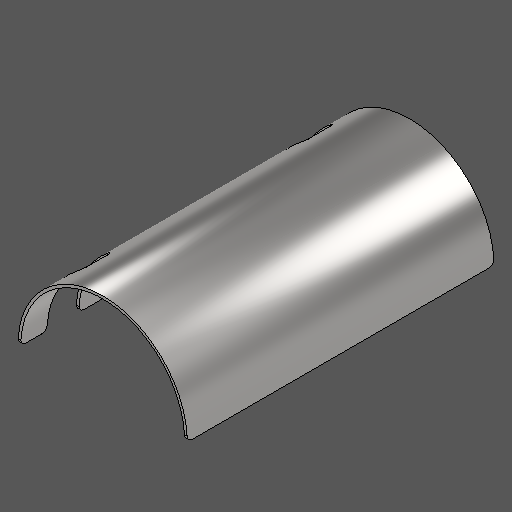
# Autodesk Inventor part: LP-screen1
Saved by Autodesk Inventor 2025 (Build 290162000, 162)
## iProperties
Created: 2024-06-04
Part Number: LP-screen1
Material: Stainless Steel
Document SubType Name: Modeling
Designer: kuzmin
Density: 8 g/cm^3
Appearance: Semi-Polished
Author: kuzmin
Autodesk Inventor part; units mm, degrees
ref_plane "YZ Plane" through (0, 0, 0) normal (1, 0, 0) x (0, 1, 0)
ref_plane "XZ Plane" through (0, 0, 0) normal (0, 1, 0) x (-1, 0, 0)
ref_plane "XY Plane" through (0, 0, 0) normal (0, 0, 1) x (1, 0, 0)
sketch "Sketch1" plane through (0, 0, 0) normal (0, 0, 1) x (1, 0, 0)
  arc A0 (16, 0) -> (-16, 0) centre (0, 0) ccw
  line L0 (-16, 0) -> (16, 0)
  dimension "d6" = 32
  constraints: 2 coincident, 2 end point, 2 point on circle, 1 centre point, 1 horizontal, 1 midpoint
  measures "d6" diameter of A0
extrude "Extrusion1" add sketch "Sketch1" along normal mid plane 58
sketch "Sketch2" plane through (0, 0, 29) normal (0, 0, 1) x (1, 0, 0)
  circle A0 centre (0, 0) radius 15.5
  arc A1 (16, 0) -> (-16, 0) centre (0, 0) ccw projected
  dimension "d3" = 0.5
  constraints: 1 centre point, 1 coincident
  measures "d3" radial gap between concentric circles of A0 A1
extrude "Extrusion2" cut sketch "Sketch2" against normal through all
sketch "Sketch3" plane through (0, 0, 0) normal (0, 1, 0) x (-1, 0, 0)
  line L0 (21, -24) -> (9, -24)
  line L1 (9, -24) -> (9, -18)
  line L2 (9, -18) -> (21, -18)
  line L3 (21, -18) -> (21, -24)
  line L4 (16, 29) -> (16, -29) projected
  line L5 (-16, -29) -> (16, -29) projected
  point P0 (0, 0)
  dimension "d7" = 7
  dimension "d8" = 5
  dimension "d9" = 6
  dimension "d10" = 12
  constraints: 8 end point, 2 parallel, 1 horizontal, 1 perpendicular, 1 other
  measures "d7" distance between parallel lines of L1 L4
  measures "d9" distance of L2.end L0.start
  measures "d10" distance of L0.start L0.end
extrude "Extrusion3" cut sketch "Sketch3" along normal through all
mirror "Mirror1" about plane through (0, 0, 0) normal (0, 0, 1) of "Extrusion3"
fillet "Fillet1" radius 1 12 edges at (-9, 12.9241, -24) (-9, 12.9241, -18) (-9, 12.9241, 18) (-9, 12.9241, 24) (-15.75, 0, 18) (-15.75, 0, 29) (-15.75, 0, 24) (-15.75, 0, -18) (-15.75, 0, -24) (-15.75, 0, -29) (15.75, 0, 29) (15.75, 0, -29)
body "Solid1"
